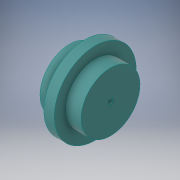
# Autodesk Inventor part: Sprocket
Saved by Autodesk Inventor 2019 (Build 230136000, 136)
## iProperties
Created: 2018-12-10
Part Number: Sprocket
Material: Generic
Document SubType Name: Modeling
Designer: scigu
Density: 1 g/cm^3
Appearance: Default
Author: scigu
Autodesk Inventor part; units mm, degrees
ref_plane "YZ Plane" through (0, 0, 0) normal (1, 0, 0) x (0, 1, 0)
ref_plane "XZ Plane" through (0, 0, 0) normal (0, 1, 0) x (-1, 0, 0)
ref_plane "XY Plane" through (0, 0, 0) normal (0, 0, 1) x (1, 0, 0)
sketch "Sketch1" plane through (0, 0, 0) normal (1, 0, 0) x (0, 1, 0)
  circle A0 centre (0, 0) radius 18
  dimension "d0" = 36
  constraints: 1 centre point, 1 coincident
  measures "d0" diameter of A0
extrude "Extrusion1" add sketch "Sketch1" along normal mid plane 25
sketch "Sketch2" plane through (0, 0, 0) normal (1, 0, 0) x (0, 1, 0)
  circle A0 centre (0, 0) radius 25
  dimension "d3" = 50
  constraints: 1 centre point, 1 coincident
  measures "d3" diameter of A0
extrude "Extrusion2" add sketch "Sketch2" along normal mid plane 6.35
sketch "Sketch3" plane through (12.5, 0, 0) normal (1, 0, 0) x (0, 0, -1)
  line L0 (-1.5, -1.5) -> (1.5, -1.5)
  line L1 (1.5, -1.5) -> (1.5, 1.5)
  line L2 (1.5, 1.5) -> (-1.5, 1.5)
  line L3 (-1.5, 1.5) -> (-1.5, -1.5)
  line L4 (-1.5, -1.5) -> (1.5, 1.5) construction
  line L5 (1.5, -1.5) -> (-1.5, 1.5) construction
  point P0 (0, 0)
  dimension "d6" = 3
  dimension "d7" = 3
  constraints: 12 end point, 2 midpoint, 2 parallel, 1 horizontal, 1 perpendicular
  measures "d6" distance of L2.end L1.end
  measures "d7" distance of L1.end L0.end
extrude "Extrusion3" cut sketch "Sketch3" against normal blind 25.4
body "Solid1"
